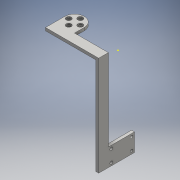
# Autodesk Inventor part: Cam_mount
Saved by Autodesk Inventor 2016 (Build 200138000, 138)
## iProperties
Created: 2016-05-11
Part Number: Cam_mount
Material: Generic
Document SubType Name: Modeling
Designer: sunilr
Density: 1 g/cm^3
Appearance: Default
Author: sunilr
Autodesk Inventor part; units mm, degrees
ref_plane "YZ Plane" through (0, 0, 0) normal (1, 0, 0) x (0, 1, 0)
ref_plane "XZ Plane" through (0, 0, 0) normal (0, 1, 0) x (-1, 0, 0)
ref_plane "XY Plane" through (0, 0, 0) normal (0, 0, 1) x (1, 0, 0)
sketch "Sketch1" plane through (0, 0, 0) normal (0, 0, 1) x (1, 0, 0)
  arc A0 (10, 0) -> (-10, 0) centre (0, 0) ccw
  line L0 (-10, 0) -> (-10, -20)
  line L1 (-10, -20) -> (10, -20)
  line L2 (10, -10) -> (10, 0)
  line L3 (10, -20) -> (45, -20)
  line L4 (45, -20) -> (45, -10)
  line L5 (45, -10) -> (10, -10)
  dimension "d1" = 20
  dimension "d2" = 35
  dimension "d3" = 10
  constraints: 12 end point, 3 perpendicular, 2 point on circle, 1 centre point, 1 coincident, 1 horizontal, 1 parallel, 1 tangent, 1 vertical
  measures "d1" distance of L0.start L0.end
  measures "d2" distance of L2.start L4.end
  measures "d3" distance of L4.end L3.end
extrude "Extrusion1" add sketch "Sketch1" along normal blind 3
sketch "Sketch2" plane through (0, 0, 0) normal (0, 0, -1) x (-1, 0, 0)
  line L0 (10, -20) -> (-45, -20) projected
  line L1 (-45, -10) -> (-10, -10) projected
  line L2 (-45, -20) -> (-42, -20)
  line L3 (-42, -20) -> (-42, -10)
  line L4 (-42, -10) -> (-45, -10)
  line L5 (-45, -10) -> (-45, -20)
  point P0 (0, 0)
  dimension "d6" = 3
  constraints: 8 end point, 2 parallel, 1 horizontal, 1 perpendicular, 1 point on line
  measures "d6" distance of L4.end L3.end
extrude "Extrusion2" add sketch "Sketch2" along normal blind 100
sketch "Sketch3" plane through (45, -20, 3) normal (1, 0, 0) x (0, 0, -1)
  point P0 (3, 20)
sketch "Sketch4" plane through (45, -20, 3) normal (1, 0, 0) x (0, 0, -1)
  point P0 (3, 20)
sketch "Sketch5" plane through (10, -10, 3) normal (0, 1, 0) x (1, 0, 0)
  line L0 (32, 3) -> (32, 103) projected
  line L1 (32, 103) -> (35, 103)
  line L2 (35, 103) -> (35, 84.5)
  line L3 (35, 84.5) -> (32, 84.5)
  line L4 (32, 84.5) -> (32, 103)
  point P0 (-10, 3)
  dimension "d9" = 3
  dimension "d10" = 18.5
  constraints: 8 end point, 2 parallel, 1 horizontal, 1 perpendicular
  measures "d9" distance of L2.end L3.end
  measures "d10" distance of L1.end L2.end
extrude "Extrusion3" add sketch "Sketch5" along normal blind 27
sketch "Sketch6" plane through (0, 0, 3) normal (0, 0, 1) x (1, 0, 0)
  point P0 (0, 0)
  point P1 (0, 6)
  point P2 (0, -6)
  point P3 (6, 0)
  point P4 (-6, 0)
hole "Hole1" at (0, 6, 3) at (0, -6, 3) at (6, 0, 3) at (-6, 0, 3) direction (0, 0, -1) diameter 4.2 end through all counterbore diameter 5.2 counterbore depth 1
sketch "Sketch7" plane through (45, -20, 3) normal (1, 0, 0) x (0, 0, -1)
  line L0 (103, 0) -> (103, 37) projected
  point P0 (3, 20)
  point P1 (100, 12.9534)
  point P2 (100, 33.9534)
  point P3 (87.5, 12.9534)
  point P4 (87.5, 33.9534)
hole "Hole2" at (45, -7.0466, -97) at (45, 13.9534, -97) at (45, -7.0466, -84.5) at (45, 13.9534, -84.5) direction (-1, 0, 0) diameter 3 end through all
body "Solid1"
